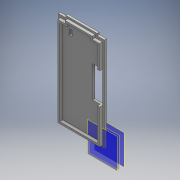
# Autodesk Inventor part: goraczesc2zotworem
Saved by Autodesk Inventor 2016 SP1 (Build 200210100, 210)
## iProperties
Created: 2019-02-21
Part Number: goraczesc2zotworem
Material: Ogólny
Document SubType Name: Modeling
Designer: Maciek
Density: 1 g/cm^3
Appearance: Domyślna
Author: Maciek
Autodesk Inventor part; units mm, degrees
ref_plane "YZ Plane" through (0, 0, 0) normal (1, 0, 0) x (0, 1, 0)
ref_plane "XZ Plane" through (0, 0, 0) normal (0, 1, 0) x (-1, 0, 0)
ref_plane "XY Plane" through (0, 0, 0) normal (0, 0, 1) x (1, 0, 0)
ref_plane "Płaszczyzna konstrukcyjna1" through (0, 19, 0) normal (0, 1, 0) x (1, 0, 0)
sketch "Szkic21" plane through (0, 19, 0) normal (0, 1, 0) x (1, 0, 0)
  line L0 (-5.3, -65.6) -> (-5.3, -67.6) projected
  line L1 (-25.3, -67.6) -> (-5.3, -67.6)
  line L2 (0, -65.6) -> (-5.3, -65.6) projected
  line L3 (-5.3, -67.6) -> (-5.3, -65.6)
  line L4 (-5.3, -65.6) -> (0, -65.6)
  line L5 (0, 0) -> (0, -65.6) projected
  line L6 (0, -65.6) -> (0, 0)
  line L7 (-30.6, -65.6) -> (-30.6, 0) projected
  line L8 (0, 0) -> (-30.6, 0)
  line L9 (-30.6, 0) -> (-30.6, -65.6)
  line L10 (-25.3, -67.6) -> (-25.3, -65.6) projected
  line L11 (-30.6, -65.6) -> (-25.3, -65.6)
  line L12 (-25.3, -65.6) -> (-25.3, -67.6)
  line L13 (-30.6, -65.6) -> (-29.1, -65.6) construction
  line L14 (-29.1, -65.6) -> (-29.1, -64.1) construction
  line L15 (-29.1, -64.1) -> (-30.6, -64.1) construction
  line L16 (-30.6, -64.1) -> (-30.6, -65.6) construction
  line L17 (-30.6, 0) -> (-29.1, 0) construction
  line L18 (-29.1, 0) -> (-29.1, -1.5) construction
  line L19 (-29.1, -1.5) -> (-30.6, -1.5) construction
  line L20 (-30.6, -1.5) -> (-30.6, 0) construction
  line L21 (0, 0) -> (-1.5, 0) construction
  line L22 (-1.5, 0) -> (-1.5, -1.5) construction
  line L23 (-1.5, -1.5) -> (0, -1.5) construction
  line L24 (0, -1.5) -> (0, 0) construction
  line L25 (0, -65.6) -> (-1.5, -65.6) construction
  line L26 (-1.5, -65.6) -> (-1.5, -64.1) construction
  line L27 (-1.5, -64.1) -> (0, -64.1) construction
  line L28 (0, -64.1) -> (0, -65.6) construction
  line L29 (-5.3, -65.6) -> (-6.8, -65.6) construction
  line L30 (-6.8, -65.6) -> (-6.8, -64.1) construction
  line L31 (-6.8, -64.1) -> (-5.3, -64.1) construction
  line L32 (-5.3, -64.1) -> (-5.3, -65.6) construction
  line L33 (-5.3, -67.6) -> (-6.8, -67.6) construction
  line L34 (-6.8, -67.6) -> (-6.8, -66.1) construction
  line L35 (-6.8, -66.1) -> (-5.3, -66.1) construction
  line L36 (-5.3, -66.1) -> (-5.3, -67.6) construction
  line L37 (-21.8, -67.6) -> (-25.3, -67.6) construction
  line L38 (-25.3, -67.6) -> (-23.8, -67.6) construction
  line L39 (-23.8, -67.6) -> (-23.8, -66.1) construction
  line L40 (-23.8, -66.1) -> (-25.3, -66.1) construction
  line L41 (-25.3, -66.1) -> (-25.3, -67.6) construction
  line L42 (-25.3, -65.6) -> (-23.8, -65.6) construction
  line L43 (-23.8, -65.6) -> (-23.8, -64.1) construction
  line L44 (-23.8, -64.1) -> (-25.3, -64.1) construction
  line L45 (-25.3, -64.1) -> (-25.3, -65.6) construction
  line L46 (-29.1, -64.1) -> (-29.1, -1.5)
  line L47 (-29.1, -1.5) -> (-1.5, -1.5)
  line L48 (-1.5, -1.5) -> (-1.5, -64.1)
  line L49 (-1.5, -64.1) -> (-6.8, -64.1)
  line L50 (-6.8, -64.1) -> (-6.8, -66.1)
  line L51 (-6.8, -66.1) -> (-23.8, -66.1)
  line L52 (-23.8, -66.1) -> (-23.8, -64.1)
  line L53 (-23.8, -64.1) -> (-29.1, -64.1)
  dimension "d115" = 1.5
  dimension "d116" = 1.5
  dimension "d117" = 1.5
  dimension "d118" = 1.5
  dimension "d119" = 1.5
  dimension "d120" = 1.5
  dimension "d121" = 1.5
  dimension "d122" = 1.5
  dimension "d123" = 1.5
  dimension "d124" = 1.5
  dimension "d125" = 1.5
  dimension "d126" = 1.5
  dimension "d127" = 1.5
  dimension "d128" = 1.5
  dimension "d129" = 1.5
  dimension "d130" = 1.5
  constraints: 96 end point, 18 equal length, 13 perpendicular, 9 horizontal
  measures "d115" distance of L15.end L14.end
  measures "d116" distance of L14.end L13.end
  measures "d117" distance of L18.end L19.end
  measures "d118" distance of L17.end L18.end
  measures "d119" distance of L23.end L22.end
  measures "d120" distance of L22.end L21.end
  measures "d121" distance of L26.end L27.end
  measures "d122" distance of L25.end L26.end
  measures "d123" distance of L30.end L31.end
  measures "d124" distance of L29.end L30.end
  measures "d125" distance of L34.end L35.end
  measures "d126" distance of L33.end L34.end
  measures "d127" distance of L40.end L39.end
  measures "d128" distance of L39.end L38.end
  measures "d129" distance of L44.end L43.end
  measures "d130" distance of L43.end L42.end
extrude "Wyciągnięcie proste19" add sketch "Szkic21" against normal blind 2
ref_plane "Płaszczyzna konstrukcyjna3" through (0, 19, 0) normal (0, 1, 0) x (1, 0, 0)
sketch "Szkic22" plane through (0, 19, 0) normal (0, 1, 0) x (1, 0, 0)
  line L0 (1.5, -67.6) -> (1.5, 1.5) projected
  line L1 (1.5, -67.6) -> (1.5, 1.5)
  line L2 (1.5, 1.5) -> (-32.1, 1.5) projected
  line L3 (1.5, 1.5) -> (-32.1, 1.5)
  line L4 (-32.1, -67.6) -> (-26.8, -67.6) projected
  line L5 (-32.1, 1.5) -> (-32.1, -67.6)
  line L6 (-32.1, -67.6) -> (-26.8, -67.6)
  line L7 (-26.8, -69.1) -> (-23.3, -69.1) projected
  line L8 (-26.8, -67.6) -> (-26.8, -69.1)
  line L9 (-7.3, -69.1) -> (-3.8, -69.1) projected
  line L10 (-26.8, -69.1) -> (-3.8, -69.1)
  line L11 (-3.8, -69.1) -> (-3.8, -67.6)
  line L12 (-3.8, -67.6) -> (1.5, -67.6) projected
  line L13 (-3.8, -67.6) -> (1.5, -67.6)
  point P0 (0, 0)
  constraints: 16 end point, 6 perpendicular, 1 collinear, 1 point on line, 1 vertical
extrude "Wyciągnięcie proste20" add sketch "Szkic22" along normal blind 1.5
ref_plane "Płaszczyzna konstrukcyjna2" through (0, 24, 0) normal (0, 1, 0) x (1, 0, 0)
ref_plane "Płaszczyzna konstrukcyjna5" through (0, 24, 0) normal (0, 1, 0) x (1, 0, 0)
ref_plane "Płaszczyzna konstrukcyjna6" through (0, 24, 0) normal (0, 1, 0) x (1, 0, 0)
ref_plane "Płaszczyzna konstrukcyjna4" through (0, 20.5, 0) normal (0, 1, 0) x (1, 0, 0)
sketch "Szkic26" plane through (0, 20.5, 0) normal (0, 1, 0) x (1, 0, 0)
  line L0 (1.5, -67.6) -> (1.5, 1.5) construction
  line L1 (1.5, 1.5) -> (1.5, -0.3) construction
  line L2 (1.5, -0.3) -> (1.5, -25.3) construction
  line L3 (1.5, -0.3) -> (1.5, -48.3) construction
  line L4 (1.5, -48.3) -> (0, -48.3) construction
  line L5 (0, -48.3) -> (-7, -48.3)
  line L6 (-7, -48.3) -> (-7, -25.3)
  line L7 (-7, -25.3) -> (0, -25.3)
  line L8 (0, -25.3) -> (0, -48.3)
  point P0 (0, 0)
  dimension "d146" = 1.8
  dimension "d147" = 25
  dimension "d148" = 48
  dimension "d149" = 7
  constraints: 16 end point, 3 point on line, 2 horizontal, 2 parallel, 1 perpendicular
  measures "d146" distance of L0.end L1.end
  measures "d147" distance of L1.end L2.end
  measures "d148" distance of L1.end L3.end
  measures "d149" distance of L6.end L7.end
extrude "Wyciągnięcie proste24" cut sketch "Szkic26" against normal blind 5
sketch "Szkic28" plane through (0, 20.5, 0) normal (0, 1, 0) x (1, 0, 0)
  line L0 (-32.1, -67.6) -> (-26.8, -67.6) construction
  line L1 (-32.1, -67.6) -> (-24.1, -67.6) construction
  line L2 (-24.1, -67.6) -> (-22.1, -67.6) construction
  line L3 (-23.3, -67.6) -> (-7.3, -67.6) construction
  line L4 (-24.1, -67.6) -> (-24.1, -69.1) construction
  line L5 (-26.8, -69.1) -> (-3.8, -69.1) construction
  line L6 (-24.1, -69.1) -> (-24.1, -62.1) construction
  line L7 (-24.1, -62.1) -> (-24.1, -58.1) construction
  line L8 (-24.1, -62.1) -> (-22.1, -62.1) construction
  line L9 (-22.1, -62.1) -> (-24.1, -62.1)
  line L10 (-24.1, -62.1) -> (-24.1, -58.1)
  line L11 (-24.1, -58.1) -> (-22.1, -58.1)
  line L12 (-22.1, -58.1) -> (-22.1, -62.1)
  point P0 (0, 0)
  dimension "d158" = 8
  dimension "d159" = 2
  dimension "d160" = 7
  dimension "d161" = 4
  dimension "d162" = 2
  constraints: 20 end point, 4 point on line, 2 horizontal, 2 parallel, 1 collinear, 1 perpendicular, 1 vertical
  measures "d158" distance of L0.start L1.end
  measures "d159" distance of L1.end L2.end
  measures "d160" distance of L4.end L6.end
  measures "d161" distance of L6.end L7.end
  measures "d162" distance of L6.end L8.end
extrude "Wyciągnięcie proste26" cut sketch "Szkic28" against normal blind 10
